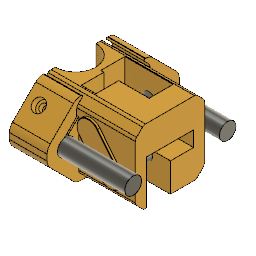
5mm_New_Y_Carriage_1.0 v10 (Autodesk Fusion 360 design; units mm, degrees)
Autodesk Fusion 360 part; units mm, degrees
sketch "スケッチ1" plane through (0, 0, 0) normal (1, 0, 0) x (0, 1, 0)
  line L0 (-17.5, 17.5) -> (17.5, 17.5)
  line L1 (17.5, 17.5) -> (31.5, 3.5)
  line L2 (31.5, 3.5) -> (31.5, -3.5)
  line L3 (31.5, -3.5) -> (17.5, -17.5)
  line L4 (17.5, -17.5) -> (-17.5, -17.5)
  line L5 (-17.5, -17.5) -> (-31.5, -3.5)
  line L6 (-31.5, -3.5) -> (-31.5, 3.5)
  line L7 (-31.5, 3.5) -> (-17.5, 17.5)
  circle A0 centre (-22.5, 0) radius 4.1
  circle A1 centre (22.5, 0) radius 4.1
  line L8 (-12.5, 17.5) -> (-16.5, 13.5)
  line L9 (-16.5, 13.5) -> (-16.5, -13.5)
  line L10 (-16.5, -13.5) -> (-12.5, -17.5)
  line L11 (12.5, 17.5) -> (16.5, 13.5)
  line L12 (16.5, 13.5) -> (16.5, -13.5)
  line L13 (16.5, -13.5) -> (12.5, -17.5)
  line L14 (-13.9142, 17.5) -> (-17.5, 13.9142)
  line L15 (-17.5, 13.9142) -> (-17.5, 9.8071)
  line L16 (-17.5, 9.8071) -> (-23.2825, 4.0246)
  line L17 (-21.8455, 4.0474) -> (-16.5, 9.3929)
  line L18 (-22.5, 0) -> (-22.5, 4.1) construction
  line L19 (-22.5, 4.1) -> (-16.5, 10.1) construction
  line L20 (-22.5, 4.1) -> (-14.0147, 4.1) construction
  line L21 (0, 17.5) -> (0, -17.5) construction
  line L22 (17.5, 9.8071) -> (23.2825, 4.0246)
  line L23 (21.8455, 4.0474) -> (16.5, 9.3929)
  line L24 (17.5, 13.9142) -> (17.5, 9.8071)
  line L25 (13.9142, 17.5) -> (17.5, 13.9142)
  line L26 (12.5, 17.5) -> (16.5, 13.5)
  dimension "d1" = 35
  dimension "d2" = 17.5
  dimension "d3" = 63
  dimension "d4" = 31.5
  dimension "d5" = 14
  dimension "d6" = 14
  dimension "d7" = 14
  dimension "d8" = 14
  dimension "d9" = 14
  dimension "d10" = 14
  dimension "d11" = 14
  dimension "d12" = 14
  dimension "d13" = 8.2
  dimension "d14" = 8.2
  dimension "d15" = 9
  dimension "d16" = 9
  dimension "d17" = 17.5
  dimension "d18" = 17.5
  dimension "d19" = 4
  dimension "d20" = 4
  dimension "d21" = 4
  dimension "d22" = 4
  dimension "d23" = 4
  dimension "d24" = 4
  dimension "d25" = 4
  dimension "d26" = 4
  dimension "d27" = 33
  dimension "d28" = 16.5
  dimension "d29" = 1
  dimension "d30" = 1
  dimension "d31" = 1
  dimension "d32" = 45
  dimension "d33" = 0.5
  dimension "d161" = 45
  constraint horizontal L0
  constraint vertical L2
  constraint horizontal L4
  constraint vertical L6
  constraint coincident L0 L8.start
  constraint perpendicular L0 L9
  constraint coincident L4 L10.end
  constraint coincident L0 L11.start
  constraint perpendicular L0 L12
  constraint coincident L4 L13.end
  constraint coincident L0 L14.start
  constraint coincident A0 L16.end
  constraint coincident A0 L17.start
  constraint coincident L9 L17.end
  constraint parallel L16 L17
  constraint parallel L8 L14
  constraint parallel L9 L15
  constraint coincident A0.centre L18.start
  constraint coincident A0 L18.end
  constraint vertical L18
  constraint coincident L9 L19.end
  constraint horizontal L20
  constraint parallel L16 L19
  constraint midpoint L0 L21.start
  constraint midpoint L4 L21.end
  constraint symmetric L8.start L21 L11.start
  constraint symmetric L8.end L21 L11.end
  constraint symmetric L14.start L21 L25.start
  constraint symmetric L14.end L21 L24.start
  constraint symmetric L15.end L21 L22.start
  constraint symmetric L16.end L21 L22.end
  constraint symmetric L17.start L21 L23.start
  constraint symmetric L17.end L21 L23.end
  measures "d1" distance of L0 L4
  measures "d2" distance of origin L0
  measures "d3" distance of L2 L6
  measures "d4" distance of origin L6
  measures "d5" distance of L0.end L2
  measures "d6" horizontal distance of L2.end L3.end
  measures "d7" horizontal distance of L0.start L6.end
  measures "d8" horizontal distance of L4.end L5.end
  measures "d9" vertical distance of L0.end L1.end
  measures "d10" vertical distance of L2.end L3.end
  measures "d11" vertical distance of L0.start L6.end
  measures "d12" vertical distance of L4.end L5.end
  measures "d13" diameter of A0
  measures "d14" diameter of A1
  measures "d15" distance of L6 A0.centre
  measures "d16" distance of L2 A1.centre
  measures "d17" distance of L0 A0.centre
  measures "d18" distance of L0 A1.centre
  measures "d19" horizontal distance of L8.start L8.end
  measures "d20" horizontal distance of L11.start L11.end
  measures "d21" horizontal distance of L12.end L13.end
  measures "d22" horizontal distance of L9.end L10.end
  measures "d23" vertical distance of L8.start L8.end
  measures "d24" vertical distance of L11.start L11.end
  measures "d25" vertical distance of L12.end L13.end
  measures "d26" vertical distance of L9.end L10.end
  measures "d27" distance of L9 L12
  measures "d28" distance of origin L9
  measures "d29" distance of L8 L14
  measures "d30" distance of L9 L15
  measures "d31" distance of L16 L17
  measures "d32" angle of L19 L20
  measures "d33" distance of L17 L19
  measures "d161" distance of A0.centre A1.centre
extrude "押し出し1" add sketch "スケッチ1" along normal blind 45 contours L0 L4 L8 L9 L10 L11 L12 L13 L26 makes body 1
extrude "押し出し2" add sketch "スケッチ1" along normal blind 18 contours L0 L4 L5 L6 L7 A0 L9 L10 L14 L15 L16 L17 | L0 L1 L2 L3 L4 A1 L12 L13 L22 L23 L24 L25 bodies 1
sketch "スケッチ2" plane through (0, 0, 17.5) normal (0, 0, 1) x (-1, 0, 0)
  line L0 (0, -12.5) -> (0, 12.5)
  line L1 (0, 12.5) -> (-45, 12.5)
  line L2 (-45, 12.5) -> (-45, -12.5)
  line L3 (-45, -12.5) -> (0, -12.5)
  line L4 (-12.27, -11) -> (-35.27, -11)
  line L5 (-35.27, -11) -> (-35.27, 0)
  line L6 (-35.27, 0) -> (-12.27, 0)
  line L7 (-12.27, 0) -> (-12.27, -11)
  line L8 (-13.77, 0) -> (-20.77, 0)
  line L9 (-20.77, 0) -> (-20.77, 11)
  line L10 (-20.77, 11) -> (-13.77, 11)
  line L11 (-13.77, 11) -> (-13.77, 0)
  circle A0 centre (0, 0) radius 9.7
  line L12 (0, -16.5) -> (-45, -16.5)
  line L13 (0, 16.5) -> (-45, 16.5)
  line L14 (-12.27, 0) -> (0, 0) construction
  line L15 (-35.27, -11) -> (-12.27, -11)
  line L16 (-12.27, -11) -> (-12.27, -11.2)
  line L17 (-12.27, -11.2) -> (-35.27, -11.2)
  line L18 (-35.27, -11.2) -> (-35.27, -11)
  line L19 (-12.27, 0) -> (-35.27, 0)
  line L20 (-35.27, 0) -> (-35.27, 0.2)
  line L21 (-35.27, 0.2) -> (-12.27, 0.2)
  line L22 (-12.27, 0.2) -> (-12.27, 0)
  dimension "d38" = 19.4
  dimension "d39" = 31.23
  dimension "d40" = 7
  dimension "d41" = 32.73
  dimension "d42" = 23
  dimension "d43" = 11
  dimension "d212" = 5.5
  dimension "d213" = 11
  dimension "d216" = 0.2
  dimension "d217" = 0.2
  constraint horizontal L4
  constraint vertical L5
  constraint horizontal L6
  constraint vertical L7
  constraint horizontal L8
  constraint vertical L9
  constraint horizontal L10
  constraint vertical L11
  constraint coincident A0.centre L14.end
  constraint collinear L6 L8
  constraint collinear L6 L14
  constraint horizontal L15
  constraint vertical L16
  constraint horizontal L17
  constraint vertical L18
  constraint collinear L7 L16
  constraint horizontal L19
  constraint vertical L20
  constraint horizontal L21
  constraint vertical L22
  measures "d38" diameter of A0
  measures "d39" distance of L2 L11
  measures "d40" distance of L9 L11
  measures "d41" distance of L2 L7
  measures "d42" distance of L5 L7
  measures "d43" distance of L4 L6
  measures "d212" distance of L4 L12
  measures "d213" distance of L8.end L9.end
  measures "d216" distance of L6 L21
  measures "d217" distance of L15 L17
extrude "押し出し3" cut sketch "スケッチ2" against normal up to surface (35 mm away) contours L0 A0 picked at (-3.2243, 0.2416) bodies 1
sketch "スケッチ3" plane through (45, 0, 0) normal (1, 0, 0) x (0, 1, 0)
  line L0 (-12.5, 17.5) -> (-16.5, 13.5)
  line L1 (-16.5, 13.5) -> (-16.5, -13.5)
  line L2 (-16.5, -13.5) -> (-12.5, -17.5)
  line L3 (-12.5, -17.5) -> (12.5, -17.5)
  line L4 (12.5, -17.5) -> (16.5, -13.5)
  line L5 (16.5, -13.5) -> (16.5, 13.5)
  line L6 (16.5, 13.5) -> (12.5, 17.5)
  line L7 (12.5, 17.5) -> (-12.5, 17.5)
  line L8 (-11, 3.635) -> (0, 3.635)
  line L9 (0, 3.635) -> (0, -17.5)
  line L10 (0, -17.5) -> (-11, -17.5)
  line L11 (-11, -17.5) -> (-11, 3.635)
  line L12 (0, 3.635) -> (11, 3.635)
  line L13 (11, 3.635) -> (11, -3.635)
  line L14 (11, -3.635) -> (0, -3.635)
  line L15 (0, -3.635) -> (0, 3.635)
  line L16 (-11, 3.635) -> (-11.2, 3.635)
  line L17 (-11.2, 3.635) -> (-11.2, -17.5)
  line L18 (-11.2, -17.5) -> (-11, -17.5)
  line L19 (-11, -17.5) -> (-11, 3.635)
  line L20 (0, 3.635) -> (0.2, 3.635)
  line L21 (0.2, 3.635) -> (0.2, -17.5)
  line L22 (0.2, -17.5) -> (0, -17.5)
  line L23 (0, -17.5) -> (0, 3.635)
  line L24 (11, 3.635) -> (11.2, 3.635)
  line L25 (11.2, 3.635) -> (11.2, -3.635)
  line L26 (11.2, -3.635) -> (11, -3.635)
  line L27 (11, -3.635) -> (11, 3.635)
  dimension "d50" = 11
  dimension "d51" = 11
  dimension "d52" = 21.135
  dimension "d53" = 7.27
  dimension "d214" = 0.2
  dimension "d215" = 0.2
  dimension "d218" = 0.2
  constraint horizontal L8
  constraint vertical L9
  constraint horizontal L10
  constraint vertical L11
  constraint coincident L3 L9.end
  constraint horizontal L12
  constraint vertical L13
  constraint horizontal L14
  constraint vertical L15
  constraint coincident origin L15
  constraint horizontal L16
  constraint vertical L17
  constraint horizontal L18
  constraint vertical L19
  constraint coincident L3 L17.end
  constraint horizontal L20
  constraint vertical L21
  constraint horizontal L22
  constraint vertical L23
  constraint coincident L3 L21.end
  constraint horizontal L24
  constraint vertical L25
  constraint horizontal L26
  constraint vertical L27
  measures "d50" distance of L9 L11
  measures "d51" distance of L9 L13
  measures "d52" distance of L8 L10
  measures "d53" distance of L12 L14
  measures "d214" distance of L9 L21
  measures "d215" distance of L17 L19
  measures "d218" distance of L13 L25
extrude "押し出し4" cut sketch "スケッチ3" against normal blind 21.04 contours L3 L11 L16 L17 L18 L19 | L3 L8 L9 L10 L11 L15 L19 L23 | L3 L9 L14 L21 L22 L23 | L9 L12 L14 L15 L20 L21 L23 bodies 1
fillet "フィレット1" radius 10 1 edges at (23.96, -5.5, 3.635) on bodies 1
extrude "押し出し5" cut sketch "スケッチ2" against normal blind 21.135 contours L4 L15 L16 L17 L18 | L4 L5 L6 L7 L8 L15 L19 | L6 L11 L19 L21 L22 | L6 L9 L19 L20 L21 | L6 L8 L9 L11 L19 L21 bodies 1
extrude "押し出し6" cut sketch "スケッチ3" against normal up to surface (9.73 mm away) contours L12 L13 L14 L21 L27 | L13 L24 L25 L26 L27 bodies 1
extrude "押し出し7" cut sketch "スケッチ2" against normal up to surface (35 mm away) contours L6 L8 L9 L11 L19 L21 | L9 L10 L11 L21 bodies 1
fillet "Fillet8" radius 8 1 edges at (12.27, 5.5, -3.635) on bodies 1
sketch "スケッチ5" plane through (0, -16.5, 0) normal (0, -1, 0) x (1, 0, 0)
  line L0 (0, 9.3929) -> (18, 9.3929)
  line L1 (18, 9.3929) -> (18, -13.5)
  line L2 (18, -13.5) -> (45, -13.5)
  line L3 (45, -13.5) -> (45, 13.5)
  line L4 (45, 13.5) -> (0, 13.5)
  line L5 (0, 13.5) -> (0, 9.3929)
  circle A0 centre (33.96, -6.365) radius 2.5
  line L6 (18, -17.5) -> (45, -17.5)
  circle A1 centre (23.77, 6.365) radius 2.5
  line L7 (0, 17.5) -> (45, 17.5)
  circle A2 centre (33.96, -6.365) radius 4
  circle A3 centre (23.77, 6.365) radius 4
  dimension "d68" = 5
  dimension "d70" = 11.04
  dimension "d71" = 11.135
  dimension "d193" = 5
  dimension "d194" = 21.23
  dimension "d195" = 11.135
  dimension "d197" = 8
  dimension "d198" = 8
  constraint concentric A0 A2
  constraint concentric A1 A3
  measures "d68" diameter of A0
  measures "d70" distance of L3 A0.centre
  measures "d71" distance of A0.centre L6
  measures "d193" diameter of A1
  measures "d194" distance of L3 A1.centre
  measures "d195" distance of A1.centre L7
  measures "d197" diameter of A2
  measures "d198" diameter of A3
extrude "Extrude41" cut sketch "スケッチ5" against normal through all contours A0 | A1 bodies 1
extrude "Extrude42" cut sketch "スケッチ5" against normal blind 1.5 contours A2 | A3 bodies 1
extrude "Extrude43" cut sketch "スケッチ5" along normal blind 1.5 from surface at -33 contours A2 | A3 bodies 1
sketch "スケッチ11" plane through (0, -17.5, 17.5) normal (0, -0.707107, 0.707107) x (1, 0, 0)
  line L0 (0, 0) -> (0, -19.799)
  line L1 (0, -19.799) -> (18, -19.799)
  line L2 (18, -19.799) -> (18, 0)
  line L3 (18, 0) -> (0, 0)
  circle A0 centre (6, -8.4099) radius 3
  circle A1 centre (6, -8.4099) radius 1.75
  line L4 (0, -24.7487) -> (18, -24.7487)
  line L5 (3, -10.142) -> (6, -11.874)
  line L6 (6, -11.874) -> (9, -10.142)
  line L7 (9, -10.142) -> (9, -6.6779)
  line L8 (9, -6.6779) -> (6, -4.9458)
  line L9 (6, -4.9458) -> (3, -6.6779)
  line L10 (3, -6.6779) -> (3, -10.142)
  point P0 (6, -8.4099)
  dimension "d113" = 6
  dimension "d114" = 3.5
  dimension "d115" = 16.3388
  dimension "d116" = 6
  dimension "d132" = 3
  constraint concentric A0 A1
  constraint coincident P0 A0.centre
  constraint parallel L0 L10
  measures "d113" diameter of A0
  measures "d114" diameter of A1
  measures "d115" distance of P0 L4
  measures "d116" distance of L0 P0
  measures "d132" distance of P0 L9
extrude "押し出し23" cut sketch "スケッチ11" against normal blind 30 contours A1 bodies 1
extrude "押し出し24" cut sketch "スケッチ11" against normal blind 3 contours A0 bodies 1
sketch "スケッチ12" plane through (0, 17.5, 17.5) normal (0, 0.707107, 0.707107) x (-1, 0, 0)
  line L0 (0, -19.799) -> (0, 0)
  line L1 (0, 0) -> (-18, 0)
  line L2 (-18, 0) -> (-18, -19.799)
  line L3 (-18, -19.799) -> (0, -19.799)
  circle A0 centre (-6, -8.4099) radius 3
  circle A1 centre (-6, -8.4099) radius 1.75
  line L4 (0, -24.7487) -> (-18, -24.7487)
  line L5 (-3, -6.6779) -> (-6, -4.9458)
  line L6 (-6, -4.9458) -> (-9, -6.6779)
  line L7 (-9, -6.6779) -> (-9, -10.142)
  line L8 (-9, -10.142) -> (-6, -11.874)
  line L9 (-6, -11.874) -> (-3, -10.142)
  line L10 (-3, -10.142) -> (-3, -6.6779)
  point P0 (-6, -8.4099)
  dimension "d121" = 6
  dimension "d122" = 3.5
  dimension "d123" = 6
  dimension "d124" = 16.3388
  dimension "d136" = 3
  constraint concentric A0 A1
  constraint coincident P0 A0.centre
  constraint parallel L0 L10
  measures "d121" diameter of A0
  measures "d122" diameter of A1
  measures "d123" distance of L0 P0
  measures "d124" distance of P0 L4
  measures "d136" distance of P0 L5
extrude "押し出し25" cut sketch "スケッチ12" against normal blind 30 contours A1 bodies 1
extrude "押し出し26" cut sketch "スケッチ12" against normal blind 3 contours A0 bodies 1
extrude "押し出し27" cut sketch "スケッチ11" against normal blind 15 from surface at -15 contours A0 | A0 L6 L7 | A0 L7 L8 | A0 L8 L9 | A0 L5 L6 | A0 L9 L10 | A0 L5 L10 | A1 bodies 1
extrude "押し出し28" cut sketch "スケッチ12" against normal blind 15 from surface at -15 contours A0 | A0 L9 L10 | A0 L5 L10 | A0 L5 L6 | A0 L8 L9 | A0 L6 L7 | A0 L7 L8 | A1 bodies 1
sketch "スケッチ14" plane through (0, 0, 0) normal (1, 0, 0) x (0, 1, 0)
  circle A0 centre (12.5, 12.5) radius 2.5
  circle A1 centre (12.5, 12.5) radius 2.35
  circle A2 centre (12.5, 12.5) radius 1.6
  dimension "d140" = 5
  dimension "d141" = 4.7
  dimension "d142" = 3.2
  dimension "d143" = 12.5
  dimension "d144" = 12.5
  constraint concentric A0 A1
  constraint concentric A1 A2
  measures "d140" diameter of A0
  measures "d141" diameter of A1
  measures "d142" diameter of A2
  measures "d143" horizontal distance of origin A0.centre
  measures "d144" vertical distance of origin A0.centre
extrude "押し出し29" cut sketch "スケッチ14" along normal blind 10 contours A2 bodies 1
extrude "押し出し30" cut sketch "スケッチ14" along normal blind 9 contours A1 bodies 1
extrude "押し出し31" cut sketch "スケッチ14" along normal blind 0.5 contours A0 bodies 1
pattern_circular "C パターン1" count 4 over 360 about axis through (1.75, 0, 0) along (1, 0, 0) of "押し出し29", "押し出し30", "押し出し31"
sketch "Sketch23" plane through (0, 0, 17.5) normal (0, 0, 1) x (-1, 0, 0)
  line L0 (-13.77, 11) -> (-13.77, 0.2)
  line L1 (-20.77, 0.2) -> (-20.77, 11)
  line L2 (-20.77, 11) -> (-13.77, 11)
  line L3 (-35.27, -11.2) -> (-35.27, 0.2)
  line L4 (-12.27, 0.2) -> (-12.27, -11.2)
  arc A0 (0, 9.7) -> (0, -9.7) centre (0, 0) ccw
  line L5 (0, 9.7) -> (0, 12.5)
  line L6 (0, 12.5) -> (-45, 12.5)
  line L7 (-45, 12.5) -> (-45, -12.5)
  line L8 (-45, -12.5) -> (0, -12.5)
  line L9 (0, -12.5) -> (0, -9.7)
  line L10 (-13.77, 0.2) -> (-12.27, 0.2)
  line L11 (-12.27, -11.2) -> (-35.27, -11.2)
  line L12 (-35.27, 0.2) -> (-20.77, 0.2)
  dimension "d186" = 24.23
  dimension "d187" = 11.23
  measures "d186" distance of L1 L7
fillet "フィレット3" radius 5 8 edges at (9, 17.5, -17.5) (9, 31.5, -3.5) (9, 31.5, 3.5) (9, 17.5, 17.5) (9, -17.5, 17.5) (9, -31.5, 3.5) (9, -31.5, -3.5) (9, -17.5, -17.5) on bodies 1
fillet "フィレット4" radius 2 8 edges at (31.5, 12.5, -17.5) (31.5, 16.5, -13.5) (22.5, 16.5, 13.5) (22.5, 12.5, 17.5) (22.5, -12.5, 17.5) (22.5, -16.5, 13.5) (31.5, -16.5, -13.5) (31.5, -12.5, -17.5) on bodies 1
fillet "フィレット5" radius 3 2 edges at (9, 17.5, 13.9142) (9, -17.5, 13.9142) on bodies 1
fillet "フィレット6" radius 0.5 6 edges at (9, 13.9142, 17.5) (9, -13.9142, 17.5) (9, 21.8455, 4.0474) (9, 23.2825, 4.0246) (9, -23.2825, 4.0246) (9, -21.8455, 4.0474) on bodies 1
sketch "Sketch1" plane through (18, 0, 0) normal (1, 0, 0) x (0, 1, 0) in component "Rods"
  arc A0 (23.1778, 4.1293) -> (23.4192, 3.9956) centre (23.5313, 4.4829) ccw
  arc A1 (21.0564, 3.8375) -> (23.4192, 3.9956) centre (22.5, 0) ccw
  arc A2 (21.0564, 3.8375) -> (21.2339, 4.659) centre (20.8804, 4.3054) ccw
  line L0 (21.2339, 4.659) -> (16.5, 9.3929)
  line L1 (16.5, 9.3929) -> (16.5, -12.6716)
  arc A3 (15.9142, -14.0858) -> (16.5, -12.6716) centre (14.5, -12.6716) ccw
  line L2 (15.9142, -14.0858) -> (13.0858, -16.9142)
  arc A4 (11.6716, -17.5) -> (13.0858, -16.9142) centre (11.6716, -15.5) ccw
  line L3 (11.6716, -17.5) -> (15.4289, -17.5)
  arc A5 (15.4289, -17.5) -> (18.9645, -16.0355) centre (15.4289, -12.5) ccw
  line L4 (18.9645, -16.0355) -> (30.0355, -4.9645)
  arc A6 (30.0355, -4.9645) -> (31.5, -1.4289) centre (26.5, -1.4289) ccw
  line L5 (31.5, -1.4289) -> (31.5, 1.4289)
  arc A7 (31.5, 1.4289) -> (30.0355, 4.9645) centre (26.5, 1.4289) ccw
  line L6 (30.0355, 4.9645) -> (18.9645, 16.0355)
  arc A8 (18.9645, 16.0355) -> (15.4289, 17.5) centre (15.4289, 12.5) ccw
  line L7 (15.4289, 17.5) -> (15.1213, 17.5)
  arc A9 (15.1213, 17.5) -> (14.7678, 16.6464) centre (15.1213, 17) ccw
  line L8 (14.7678, 16.6464) -> (16.6213, 14.7929)
  arc A10 (17.5, 12.6716) -> (16.6213, 14.7929) centre (14.5, 12.6716) ccw
  line L9 (17.5, 12.6716) -> (17.5, 9.8071)
  line L10 (17.5, 9.8071) -> (23.1778, 4.1293)
  circle A11 centre (22.5, 0) radius 4
  arc A12 (-23.4192, 3.9956) -> (-21.0564, 3.8375) centre (-22.5, 0) ccw
  circle A13 centre (-22.5, 0) radius 4
  dimension "d219" = 8
  dimension "d220" = 8
  constraint concentric A1 A11
  constraint concentric A12 A13
  measures "d219" diameter of A11
  measures "d220" diameter of A13
extrude "Extrude1" add sketch "Sketch1" along normal blind 50 from surface at -18 separate body contours A11 | A13 makes body 2 at (16.6667, -18.5199, -0.3983) makes body 3 at (16.6667, 26.4801, -0.3983) in component "Rods"
sketch "Sketch1 (2)" plane through (0, -16.5, 0) normal (0, -1, 0) x (1, 0, 0) in component "Pin"
  circle A0 centre (33.96, -6.365) radius 4
  circle A1 centre (23.77, 6.365) radius 4
  line L0 (18, -12.6716) -> (45, -12.6716)
  line L1 (45, -12.6716) -> (45, 12.6716)
  line L2 (45, 12.6716) -> (0, 12.6716)
  line L3 (0, 12.6716) -> (0, 9.3929)
  line L4 (0, 9.3929) -> (18, 9.3929)
  line L5 (18, 9.3929) -> (18, -12.6716)
  circle A2 centre (23.77, 6.365) radius 3.5
  circle A3 centre (23.77, 6.365) radius 2.5
  circle A4 centre (33.96, -6.365) radius 2.5
  circle A5 centre (33.96, -6.365) radius 3.5
  dimension "d204" = 7
  dimension "d205" = 5
  dimension "d206" = 5
  dimension "d207" = 7
  constraint concentric A1 A2
  constraint concentric A2 A3
  constraint concentric A0 A4
  constraint concentric A4 A5
  measures "d204" diameter of A2
  measures "d205" diameter of A3
  measures "d206" diameter of A4
  measures "d207" diameter of A5
extrude "Extrude1'" add sketch "Sketch1 (2)" against normal blind 1.5 separate body contours A2 | A3 | A4 | A5 makes body 4 at (24.0219, -16.5, 7.451) makes body 5 at (32.0659, -16.5, -5.7317) in component "Pin"
extrude "Extrude2" add sketch "Sketch1 (2)" against normal up to surface (33 mm away) contours A3 | A4 bodies 4 5 in component "Pin"
sketch "Sketch1 (3)" plane through (0, -16.5, 0) normal (0, -1, 0) x (1, 0, 0) in component "Cover"
  circle A0 centre (33.96, -6.365) radius 4
  circle A1 centre (23.77, 6.365) radius 4
  line L0 (18, -12.6716) -> (45, -12.6716)
  line L1 (45, -12.6716) -> (45, 12.6716)
  line L2 (45, 12.6716) -> (0, 12.6716)
  line L3 (0, 12.6716) -> (0, 9.3929)
  line L4 (0, 9.3929) -> (18, 9.3929)
  line L5 (18, 9.3929) -> (18, -12.6716)
  circle A2 centre (23.77, 6.365) radius 5.5
  circle A3 centre (33.96, -6.365) radius 5.5
  line L6 (28.0638, 9.8021) -> (38.2538, -2.9279)
  line L7 (19.4762, 2.9279) -> (29.6662, -9.8021)
  dimension "d224" = 11
  dimension "d228" = 11
  constraint concentric A1 A2
  constraint concentric A0 A3
  constraint coincident A2 L6.start
  constraint coincident A3 L6.end
  constraint tangent A3 L6
  constraint coincident A2 L7.start
  constraint coincident A3 L7.end
  constraint tangent A3 L7
  constraint tangent A2 L6
  constraint tangent A2 L7
  measures "d224" diameter of A2
  measures "d228" diameter of A3
extrude "Extrude1''" add sketch "Sketch1 (3)" along normal blind 1.2 separate body contours A0 | A1 | A2 | A2 A3 L6 L7 | A3 makes body 6 in component "Cover"
chamfer "Chamfer1" distance 0.2 angle 45 4 edges at (20.3329, -17.7, 10.6588) (24.5712, -17.7, -3.4371) (37.3971, -17.7, -10.6588) (33.1588, -17.7, 3.4371) on bodies 6 in component "Cover"
component "Rods" placed x (1, 0, 0) y (0, 1, 0) z (0, 0, 1) at (0, 0, 0)
component "Pin" placed x (1, 0, 0) y (0, 1, 0) z (0, 0, 1) at (0, 0, 0)
component "Cover" placed x (1, 0, 0) y (0, 1, 0) z (0, 0, 1) at (0, 0, 0)
equation "d2 = d1 / 2"
equation "d4 = d3 / 2"
equation "d9 = d5"
equation "d10 = d6"
equation "d11 = d7"
equation "d12 = d8"
equation "d13 = 8.4 mm - 0.2 mm"
equation "d14 = 8.4 mm - 0.2 mm"
equation "d17 = d2"
equation "d18 = d2"
equation "d23 = d19"
equation "d24 = d20"
equation "d25 = d21"
equation "d26 = d22"
equation "d28 = d27 / 2"
equation "d33 = d31 / 2"
equation "d39 = 32.5 mm - 1.27 mm - 1.5 mm + 1.5 mm"
equation "d40 = 5.5 mm + 1.5 mm"
equation "d41 = d39 + 1.5 mm"
equation "d54 = -19.77 mm - 1.27 mm"
equation "d70 = 9.77 mm + 1.27 mm"
equation "d193 = d68"
equation "d198 = d197"
equation "d215 = d214"
equation "d217 = d216"
equation "d218 = d214"
equation "d228 = d224"
